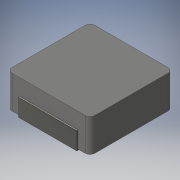
# Autodesk Inventor part: SRP1770TA-101M
Saved by Autodesk Inventor 2016 (Build 200138000, 138)
## iProperties
Created: 2016-08-10
Part Number: SRP1770TA-101M
Material: Generic
Document SubType Name: Modeling
Designer: jfixelle
Density: 1 g/cm^3
Appearance: Gray
Author: jfixelle
Autodesk Inventor part; units mm, degrees
ref_plane "YZ Plane" through (0, 0, 0) normal (1, 0, 0) x (0, 1, 0)
ref_plane "XZ Plane" through (0, 0, 0) normal (0, 1, 0) x (-1, 0, 0)
ref_plane "XY Plane" through (0, 0, 0) normal (0, 0, 1) x (1, 0, 0)
sketch "Sketch1" plane through (0, 0, 0) normal (0, 1, 0) x (-1, 0, 0)
  line L0 (8.45, 8.45) -> (-8.45, 8.45)
  line L1 (-8.45, 8.45) -> (-8.45, -8.45)
  line L2 (-8.45, -8.45) -> (8.45, -8.45)
  line L3 (8.45, -8.45) -> (8.45, 8.45)
  point P0 (0, 0)
  dimension "d0" = 16.9
  dimension "d1" = 16.9
  dimension "d2" = 8.45
  dimension "d3" = 8.45
  constraints: 8 end point, 2 parallel, 1 horizontal, 1 perpendicular
  measures "d0" distance of L2.end L0.start
  measures "d1" distance of L1.end L2.end
  measures "d2" distance from line of point (0, 0) L3
  measures "d3" distance from line of point (0, 0) L2
extrude "Extrusion1" add sketch "Sketch1" along normal blind 6.7
fillet "Fillet1" radius 1 4 edges at (8.45, 3.35, -8.45) (8.45, 3.35, 8.45) (-8.45, 3.35, 8.45) (-8.45, 3.35, -8.45)
sketch "Sketch2" plane through (0, 0, 0) normal (0, -1, 0) x (1, 0, 0)
  line L0 (5.95, 8.65) -> (-5.95, 8.65)
  line L1 (-5.95, 8.65) -> (-5.95, 6.55)
  line L2 (-5.95, 6.55) -> (5.95, 6.55)
  line L3 (5.95, 6.55) -> (5.95, 8.65)
  point P0 (0, 0)
  dimension "d7" = 11.9
  dimension "d8" = 5.95
  dimension "d9" = 2.1
  dimension "d10" = 8.65
  constraints: 8 end point, 2 parallel, 1 horizontal, 1 perpendicular
  measures "d7" distance of L0.start L0.end
  measures "d8" distance from line of point (0, 0) L3
  measures "d9" distance of L2.end L0.start
  measures "d10" distance from line of point (0, 0) L0
extrude "Extrusion2" add sketch "Sketch2" along normal blind 0.25 and the other way blind 3.35
mirror "Mirror1" about plane through (0, 0, 0) normal (0, 0, 1) of "Extrusion2"
body "Solid1"
